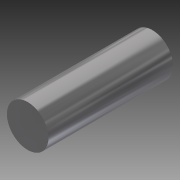
# Autodesk Inventor part: Gearmotor_Shaft
Saved by Autodesk Inventor 2013 (Build 170138000, 138)
## iProperties
Created: 2015-07-02
Part Number: Gearmotor_Shaft
Material: Steel, Carbon
Document SubType Name: Modeling
Designer: Kyle
Density: 7.87 g/cm^3
Mass: 0.499267 g
Surface Area: 0.987755 cm^2
Volume: 0.0634393 cm^3
Author: Kyle
Autodesk Inventor part; units mm, degrees
ref_plane "YZ Plane" through (0, 0, 0) normal (1, 0, 0) x (0, 1, 0)
ref_plane "XZ Plane" through (0, 0, 0) normal (0, 1, 0) x (-1, 0, 0)
ref_plane "XY Plane" through (0, 0, 0) normal (0, 0, 1) x (1, 0, 0)
sketch "Sketch1" plane through (0, 0, 0) normal (0, 0, 1) x (1, 0, 0)
  circle A0 centre (0, 0) radius 1.4986
  dimension "d0" = 2.9972
  constraints: 1 centre point, 1 coincident
  measures "d0" diameter of A0
extrude "Extrusion1" add sketch "Sketch1" along normal blind 8.9916
body "Solid1"
